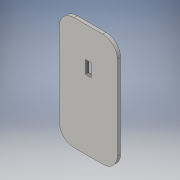
# Autodesk Inventor part: RTS gift base
Saved by Autodesk Inventor 2016 (Build 200138000, 138)
## iProperties
Created: 2017-12-18
Part Number: RTS gift base
Material: Generic
Document SubType Name: Modeling
Designer: student
Density: 1 g/cm^3
Appearance: Default
Author: student
Autodesk Inventor part; units mm, degrees
ref_plane "YZ Plane" through (0, 0, 0) normal (1, 0, 0) x (0, 1, 0)
ref_plane "XZ Plane" through (0, 0, 0) normal (0, 1, 0) x (-1, 0, 0)
ref_plane "XY Plane" through (0, 0, 0) normal (0, 0, 1) x (1, 0, 0)
sketch "Sketch1" plane through (0, 0, 0) normal (0, 0, 1) x (1, 0, 0)
  line L0 (22.86, 44.45) -> (-22.86, 44.45)
  line L1 (-22.86, 44.45) -> (-22.86, -44.45)
  line L2 (-22.86, -44.45) -> (22.86, -44.45)
  line L3 (22.86, -44.45) -> (22.86, 44.45)
  line L4 (22.86, 44.45) -> (-22.86, -44.45) construction
  line L5 (-22.86, 44.45) -> (22.86, -44.45) construction
  line L6 (-2.2225, 20.3972) -> (2.2225, 20.3972)
  line L7 (2.2225, 20.3972) -> (2.2225, 10.2372)
  line L8 (2.2225, 10.2372) -> (-2.2225, 10.2372)
  line L9 (-2.2225, 10.2372) -> (-2.2225, 20.3972)
  line L10 (-2.2225, 20.3972) -> (2.2225, 10.2372) construction
  line L11 (2.2225, 20.3972) -> (-2.2225, 10.2372) construction
  dimension "d0" = 45.72
  dimension "d1" = 88.9
  dimension "d15" = 10.16
  constraints: 24 end point, 4 parallel, 2 horizontal, 2 perpendicular
  measures "d0" distance of L2.end L1.end
  measures "d1" distance of L1.end L0.end
  measures "d15" distance of L7.start L7.end
extrude "Extrusion3" add sketch "Sketch1" along normal blind 2.54
fillet "Fillet3" radius 11.43 4 edges at (22.86, 44.45, 1.27) (22.86, -44.45, 1.27) (-22.86, -44.45, 1.27) (-22.86, 44.45, 1.27)
body "Solid3"
